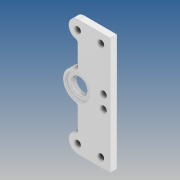
# Autodesk Inventor part: 2113_Nut Stop Plate_V1
Saved by Autodesk Inventor 2020 (Build 240168000, 168)
## iProperties
Created: 2019-11-08
Part Number: 2113_Nut Stop Plate_V1
Material: ABS Plastic
Document SubType Name: Modeling
Designer: RFLab
Density: 1.06 g/cm^3
Appearance: Smooth - White
Author: RFLab
Autodesk Inventor part; units mm, degrees
ref_plane "YZ Plane" through (0, 0, 0) normal (1, 0, 0) x (0, 1, 0)
ref_plane "XZ Plane" through (0, 0, 0) normal (0, 1, 0) x (-1, 0, 0)
ref_plane "XY Plane" through (0, 0, 0) normal (0, 0, 1) x (1, 0, 0)
sketch "Sketch1" plane through (0, 0, 0) normal (0, 0, 1) x (1, 0, 0)
  circle A0 centre (0, 0) radius 20
  line L0 (-25, -45) -> (25, -45)
  line L1 (25, -45) -> (25, 45)
  line L2 (25, 45) -> (-25, 45)
  line L3 (-25, 45) -> (-25, -45)
  point P0 (-20, 0)
  point P1 (20, 0)
  dimension "d0" = 40
  dimension "d17" = 90
  dimension "d18" = 50
  dimension "d19" = 25
  dimension "d20" = 45
  constraints: 8 end point, 2 parallel, 1 centre point, 1 coincident, 1 horizontal, 1 perpendicular
  measures "d0" diameter of A0
  measures "d17" distance of L2.end L0.start
  measures "d18" distance of L1.end L2.end
  measures "d19" distance from line of L3 point (0, 0)
  measures "d20" distance from line of L2 point (0, 0)
extrude "Extrusion1" add sketch "Sketch1" along normal blind 5 contours A0 | L3 L2 L1 L0
sketch "Sketch2" plane through (0, 0, 5) normal (0, 0, 1) x (1, 0, 0)
  line L0 (-25, 45) -> (-25, -45) projected
  line L1 (25, 45) -> (-25, 45) projected
  circle A0 centre (0, 0) radius 6.3
  dimension "d37" = 12.6
  constraints: 1 centre point, 1 coincident
  measures "d37" diameter of A0
extrude "Extrusion2" cut sketch "Sketch2" against normal blind 5 from surface at 0
sketch "Sketch3" plane through (0, 0, 5) normal (0, 0, 1) x (1, 0, 0)
  circle A0 centre (0, 0) radius 4.5 projected
  circle A1 centre (0, 0) radius 9.4
  dimension "d6" = 18.8
  constraints: 1 centre point, 1 coincident
  measures "d6" diameter of A1
extrude "Extrusion3" cut sketch "Sketch3" against normal blind 1.1
fillet "Fillet1" radius 0.2 1 edges at (-9.4, 0, 3.9)
sketch "Sketch4" plane through (0, 0, 0) normal (0, 0, -1) x (-1, 0, 0)
  circle A0 centre (18, 38) radius 2.3
  circle A1 centre (-18, 38) radius 2.3
  circle A2 centre (18, -38) radius 2.3
  circle A3 centre (-18, -38) radius 2.3
  line L0 (-25, 45) -> (25, 45) projected
  line L1 (25, -45) -> (-25, -45) projected
  line L2 (25, 45) -> (25, -45) projected
  line L3 (-25, -45) -> (-25, 45) projected
  circle A4 centre (-20, 5) radius 2.3
  circle A5 centre (-20, -5) radius 2.3
  line L4 (-20, 5) -> (-20, -5)
  circle A6 centre (0, 0) radius 6.3 projected
  circle A7 centre (0, 0) radius 11.3
  line L5 (0, 45) -> (0, 11.3) construction
  line L6 (0, -11.3) -> (0, -45) construction
  circle A8 centre (0, 38) radius 2.3
  circle A9 centre (0, -38) radius 2.3
  arc A10 (0, 31) -> (0, 45) centre (0, 38) ccw
  arc A11 (0, -45) -> (0, -31) centre (0, -38) ccw
  line L7 (0, 31) -> (0, 11.3)
  line L8 (0, -11.3) -> (0, -31)
  point P0 (-20, 0)
  dimension "d10" = 4.6
  dimension "d21" = 7
  dimension "d22" = 7
  dimension "d23" = 7
  dimension "d24" = 7
  dimension "d25" = 7
  dimension "d26" = 7
  dimension "d27" = 7
  dimension "d28" = 7
  dimension "d32" = 10
  dimension "d34" = 5
  dimension "d35" = 5
  dimension "d38" = 90
  dimension "d39" = 5
  dimension "d40" = 4.6
  dimension "d41" = 4.6
  constraints: 11 centre point, 10 end point, 6 point on circle, 5 equal radius, 5 point on line, 3 horizontal alignment, 3 midpoint, 2 coincident, 1 collinear, 1 tangent, 1 vertical
  measures "d10" diameter of A0
  measures "d21" distance from line of L0 A0.centre
  measures "d22" distance from line of L0 A1.centre
  measures "d23" distance from line of L1 A2.centre
  measures "d24" distance from line of L2 A2.centre
  measures "d25" distance from line of L2 A0.centre
  measures "d26" distance from line of L3 A1.centre
  measures "d27" distance from line of L1 A3.centre
  measures "d28" distance from line of L3 A3.centre
  measures "d32" distance of L4.end L4.start
  measures "d34" distance from line of L3 L4.start
  measures "d35" distance from line of L3 L4.end
  measures "d38" distance of L0.end L1.start
  measures "d39" radial gap between concentric circles of A6 A7
  measures "d40" diameter of A8
  measures "d41" diameter of A9
extrude "Extrusion4" cut sketch "Sketch4" against normal through all contours A0 | A1 | A2 | A3 | L0 L2 L1 A11 L8 A7 L7 A10 | A4 | A5 | A8 | A9
fillet "Fillet3" radius 2 4 edges at (0, 31, 2.5) (0, 11.3, 2.5) (0, -11.3, 2.5) (0, -31, 2.5)
equation "\"d19\" = 0.5 * d18"
equation "\"d20\" = 0.5 * d17"
equation "\"d22\" = d21"
equation "\"d23\" = d21"
equation "\"d24\" = d23"
equation "\"d26\" = d22"
equation "\"d27\" = d24"
equation "\"d28\" = d24"
equation "\"d40\" = d10"
equation "\"d41\" = d10"
body "Solid1"
